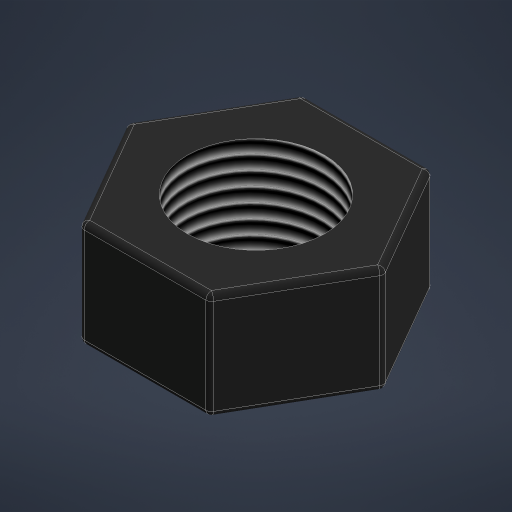
# Autodesk Inventor part: M5 Nut
Saved by Autodesk Inventor 2024 (Build 280153000, 153)
## iProperties
Created: 2024-10-26
Part Number: M5 Nut
Material: Generic
Document SubType Name: Modeling
Designer: jerem
Density: 1 g/cm^3
Appearance: Default
Author: jerem
Autodesk Inventor part; units mm, degrees
ref_plane "YZ Plane" through (0, 0, 0) normal (1, 0, 0) x (0, 1, 0)
ref_plane "XZ Plane" through (0, 0, 0) normal (0, 1, 0) x (-1, 0, 0)
ref_plane "XY Plane" through (0, 0, 0) normal (0, 0, 1) x (1, 0, 0)
sketch "Sketch1" plane through (0, 0, 0) normal (0, 1, 0) x (-1, 0, 0)
  line L0 (4.5726, 0) -> (2.2863, -3.96)
  line L1 (2.2863, -3.96) -> (-2.2863, -3.96)
  line L2 (-2.2863, -3.96) -> (-4.5726, 0)
  line L3 (-4.5726, 0) -> (-2.2863, 3.96)
  line L4 (-2.2863, 3.96) -> (2.2863, 3.96)
  line L5 (2.2863, 3.96) -> (4.5726, 0)
  circle A0 centre (0, 0) radius 2.44
  dimension "d0" = 7.92
  dimension "d1" = 4.88
  constraints: 12 end point, 2 coincident, 1 centre point, 1 horizontal, 13 other
  measures "d0" distance between parallel lines of L4 L1
  measures "d1" diameter of A0
extrude "Extrusion1" add sketch "Sketch1" along normal blind 3.8
fillet "Fillet1" radius 0.2 18 edges at (3.4295, 3.8, 1.98) (0, 3.8, 3.96) (2.2863, 1.9, 3.96) (0, 0, 3.96) (-2.2863, 1.9, 3.96) (3.4295, 0, 1.98) (4.5726, 1.9, 0) (2.2863, 1.9, -3.96) (3.4295, 3.8, -1.98) (3.4295, 0, -1.98) (-2.2863, 1.9, -3.96) (0, 3.8, -3.96) (0, 0, -3.96) (-3.4295, 3.8, 1.98) (-3.4295, 3.8, -1.98) (-4.5726, 1.9, 0) (-3.4295, 0, -1.98) (-3.4295, 0, 1.98)
thread "Thread1" size "M5x0.5" class "6H" standard "ANSI Metric M Profile" full length
body "Solid1"
